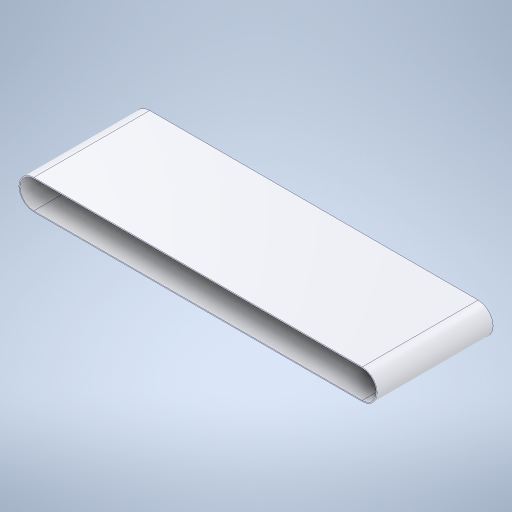
# Autodesk Inventor part: HCMUTE-CDT23-BELT_BTC
Saved by Autodesk Inventor 2023 (Build 270158000, 158)
## iProperties
Created: 2023-10-30
Part Number: HCMUTE-CDT23-BELT_BTC
Material: PVC, Unplasticized
Document SubType Name: Modeling
Designer: havie
Density: 1.29 g/cm^3
Appearance: PTFE
Mass: 463.468 g
Surface Area: 3622.72 cm^2
Volume: 359.278 cm^3
Author: havie
Autodesk Inventor part; units mm, degrees
ref_plane "YZ Plane" through (0, 0, 0) normal (1, 0, 0) x (0, 1, 0)
ref_plane "XZ Plane" through (0, 0, 0) normal (0, 1, 0) x (-1, 0, 0)
ref_plane "XY Plane" through (0, 0, 0) normal (0, 0, 1) x (1, 0, 0)
sketch "Sketch1" plane through (0, 0, 0) normal (0, 1, 0) x (-1, 0, 0)
  line L0 (370, 0) -> (-370, 0) construction
  line L1 (340, 30) -> (-340, 30)
  line L2 (-340, -30) -> (340, -30)
  arc A0 (340, -30) -> (340, 30) centre (340, 0) ccw
  arc A1 (-340, 30) -> (-340, -30) centre (-340, 0) ccw
  point P0 (0, 0)
  point P1 (0, 0)
  point P2 (-370, 0)
  point P3 (370, 0)
  dimension "d2" = 60
  dimension "d7" = 680
  constraints: 8 end point, 8 point on circle, 4 tangent, 2 centre point, 2 point on line, 1 coincident, 1 horizontal, 1 midpoint, 1 parallel
  measures "d2" distance between parallel lines of L2 L1
  measures "d7" distance of A1.centre A0.centre
ref_plane "Work Plane1" through (-340, 0, -30) normal (-1, 0, 0) x (0, -1, 0)
sketch "Sketch2" plane through (-340, 0, -30) normal (-1, 0, 0) x (0, -1, 0)
  line L0 (-120, 1) -> (120, 1)
  line L1 (120, 1) -> (120, -1)
  line L2 (120, -1) -> (-120, -1)
  line L3 (-120, -1) -> (-120, 1)
  line L4 (-120, 1) -> (120, -1) construction
  line L5 (120, 1) -> (-120, -1) construction
  line L6 (0, 60) -> (0, 0) projected
  point P0 (0, 30)
  dimension "d3" = 240
  dimension "d4" = 2
  constraints: 12 end point, 2 midpoint, 2 parallel, 1 horizontal, 1 perpendicular
  measures "d3" distance of L1.end L2.end
  measures "d4" distance of L0.end L1.end
sweep "Sweep1" add profiles "Sketch2" path "Sketch1" path curves A0 L1 A1 L2
body "Solid1"
